Autodesk Inventor part; units mm, degrees
(part 2 of 15)
  arc A531 (-9.765, -99.9538) -> (-9.765, -99.8522) centre (-9.765, -99.903) ccw
  arc A532 (-11.035, -99.8522) -> (-11.035, -99.9538) centre (-11.035, -99.903) ccw
  arc A533 (-23.984, 46.0572) -> (-23.984, 46.1588) centre (-23.984, 46.108) ccw
  line L129 (-17.235, -109.297) -> (-17.235, -106.503)
  arc A534 (-17.1842, -106.503) -> (-17.2858, -106.503) centre (-17.235, -106.503) ccw
  arc A535 (-17.2858, -109.297) -> (-17.1842, -109.297) centre (-17.235, -109.297) ccw
  line L130 (-17.235, -106.503) -> (-15.965, -106.503)
  arc A536 (-15.965, -106.5538) -> (-15.965, -106.4522) centre (-15.965, -106.503) ccw
  arc A537 (-17.235, -106.4522) -> (-17.235, -106.5538) centre (-17.235, -106.503) ccw
  line L131 (-15.965, -106.503) -> (-15.965, -109.297)
  arc A538 (-16.0158, -109.297) -> (-15.9142, -109.297) centre (-15.965, -109.297) ccw
  arc A539 (-15.9142, -106.503) -> (-16.0158, -106.503) centre (-15.965, -106.503) ccw
  line L132 (-15.965, -109.297) -> (-17.235, -109.297)
  arc A540 (-17.235, -109.2462) -> (-17.235, -109.3478) centre (-17.235, -109.297) ccw
  arc A541 (-15.965, -109.3478) -> (-15.965, -109.2462) centre (-15.965, -109.297) ccw
  arc A542 (-26.016, 46.1588) -> (-26.016, 46.0572) centre (-26.016, 46.108) ccw
  line L133 (-15.808, -109.416) -> (-15.808, -107.384)
  arc A543 (-15.7572, -107.384) -> (-15.8588, -107.384) centre (-15.808, -107.384) ccw
  arc A544 (-15.8588, -109.416) -> (-15.7572, -109.416) centre (-15.808, -109.416) ccw
  line L134 (-15.808, -107.384) -> (-14.792, -107.384)
  arc A545 (-14.792, -107.4348) -> (-14.792, -107.3332) centre (-14.792, -107.384) ccw
  arc A546 (-15.808, -107.3332) -> (-15.808, -107.4348) centre (-15.808, -107.384) ccw
  line L135 (-14.792, -107.384) -> (-14.792, -109.416)
  arc A547 (-14.8428, -109.416) -> (-14.7412, -109.416) centre (-14.792, -109.416) ccw
  arc A548 (-14.7412, -107.384) -> (-14.8428, -107.384) centre (-14.792, -107.384) ccw
  line L136 (-14.792, -109.416) -> (-15.808, -109.416)
  arc A549 (-15.808, -109.3652) -> (-15.808, -109.4668) centre (-15.808, -109.416) ccw
  arc A550 (-14.792, -109.4668) -> (-14.792, -109.3652) centre (-14.792, -109.416) ccw
  line L137 (-23.984, 46.108) -> (-23.984, 45.092)
  line L138 (9.757, -79.0892) -> (9.757, -74.1108)
  arc A551 (9.8078, -74.1108) -> (9.7062, -74.1108) centre (9.757, -74.1108) ccw
  arc A552 (9.7062, -79.0892) -> (9.8078, -79.0892) centre (9.757, -79.0892) ccw
  line L139 (9.757, -74.1108) -> (12.043, -74.1108)
  arc A553 (12.043, -74.1616) -> (12.043, -74.06) centre (12.043, -74.1108) ccw
  arc A554 (9.757, -74.06) -> (9.757, -74.1616) centre (9.757, -74.1108) ccw
  line L140 (12.043, -74.1108) -> (12.043, -79.0892)
  arc A555 (11.9922, -79.0892) -> (12.0938, -79.0892) centre (12.043, -79.0892) ccw
  arc A556 (12.0938, -74.1108) -> (11.9922, -74.1108) centre (12.043, -74.1108) ccw
  line L141 (12.043, -79.0892) -> (9.757, -79.0892)
  arc A557 (9.757, -79.0384) -> (9.757, -79.14) centre (9.757, -79.0892) ccw
  arc A558 (12.043, -79.14) -> (12.043, -79.0384) centre (12.043, -79.0892) ccw
  arc A559 (-24.0348, 45.092) -> (-23.9332, 45.092) centre (-23.984, 45.092) ccw
  line L142 (9.203, -79.065) -> (11.997, -79.065)
  arc A560 (11.997, -79.1158) -> (11.997, -79.0142) centre (11.997, -79.065) ccw
  arc A561 (9.203, -79.0142) -> (9.203, -79.1158) centre (9.203, -79.065) ccw
  line L143 (11.997, -79.065) -> (11.997, -80.335)
  arc A562 (11.9462, -80.335) -> (12.0478, -80.335) centre (11.997, -80.335) ccw
  arc A563 (12.0478, -79.065) -> (11.9462, -79.065) centre (11.997, -79.065) ccw
  line L144 (11.997, -80.335) -> (9.203, -80.335)
  arc A564 (9.203, -80.2842) -> (9.203, -80.3858) centre (9.203, -80.335) ccw
  arc A565 (11.997, -80.3858) -> (11.997, -80.2842) centre (11.997, -80.335) ccw
  line L145 (9.203, -80.335) -> (9.203, -79.065)
  arc A566 (9.2538, -79.065) -> (9.1522, -79.065) centre (9.203, -79.065) ccw
  arc A567 (9.1522, -80.335) -> (9.2538, -80.335) centre (9.203, -80.335) ccw
  arc A568 (-23.9332, 46.108) -> (-24.0348, 46.108) centre (-23.984, 46.108) ccw
  line L146 (8.165, -77.997) -> (8.165, -75.203)
  arc A569 (8.2158, -75.203) -> (8.1142, -75.203) centre (8.165, -75.203) ccw
  arc A570 (8.1142, -77.997) -> (8.2158, -77.997) centre (8.165, -77.997) ccw
  line L147 (8.165, -75.203) -> (9.435, -75.203)
  arc A571 (9.435, -75.2538) -> (9.435, -75.1522) centre (9.435, -75.203) ccw
  arc A572 (8.165, -75.1522) -> (8.165, -75.2538) centre (8.165, -75.203) ccw
  line L148 (9.435, -75.203) -> (9.435, -77.997)
  arc A573 (9.3842, -77.997) -> (9.4858, -77.997) centre (9.435, -77.997) ccw
  arc A574 (9.4858, -75.203) -> (9.3842, -75.203) centre (9.435, -75.203) ccw
  line L149 (9.435, -77.997) -> (8.165, -77.997)
  arc A575 (8.165, -77.9462) -> (8.165, -78.0478) centre (8.165, -77.997) ccw
  arc A576 (9.435, -78.0478) -> (9.435, -77.9462) centre (9.435, -77.997) ccw
  line L150 (-23.984, 45.092) -> (-26.016, 45.092)
  line L151 (9.584, -83.992) -> (11.616, -83.992)
  arc A577 (11.616, -84.0428) -> (11.616, -83.9412) centre (11.616, -83.992) ccw
  arc A578 (9.584, -83.9412) -> (9.584, -84.0428) centre (9.584, -83.992) ccw
  line L152 (11.616, -83.992) -> (11.616, -85.008)
  arc A579 (11.5652, -85.008) -> (11.6668, -85.008) centre (11.616, -85.008) ccw
  arc A580 (11.6668, -83.992) -> (11.5652, -83.992) centre (11.616, -83.992) ccw
  line L153 (11.616, -85.008) -> (9.584, -85.008)
  arc A581 (9.584, -84.9572) -> (9.584, -85.0588) centre (9.584, -85.008) ccw
  arc A582 (11.616, -85.0588) -> (11.616, -84.9572) centre (11.616, -85.008) ccw
  line L154 (9.584, -85.008) -> (9.584, -83.992)
  arc A583 (9.6348, -83.992) -> (9.5332, -83.992) centre (9.584, -83.992) ccw
  arc A584 (9.5332, -85.008) -> (9.6348, -85.008) centre (9.584, -85.008) ccw
  arc A585 (-26.016, 45.1428) -> (-26.016, 45.0412) centre (-26.016, 45.092) ccw
  line L155 (12.365, -77.997) -> (12.365, -75.203)
  arc A586 (12.4158, -75.203) -> (12.3142, -75.203) centre (12.365, -75.203) ccw
  arc A587 (12.3142, -77.997) -> (12.4158, -77.997) centre (12.365, -77.997) ccw
  line L156 (12.365, -75.203) -> (13.635, -75.203)
  arc A588 (13.635, -75.2538) -> (13.635, -75.1522) centre (13.635, -75.203) ccw
  arc A589 (12.365, -75.1522) -> (12.365, -75.2538) centre (12.365, -75.203) ccw
  line L157 (13.635, -75.203) -> (13.635, -77.997)
  arc A590 (13.5842, -77.997) -> (13.6858, -77.997) centre (13.635, -77.997) ccw
  arc A591 (13.6858, -75.203) -> (13.5842, -75.203) centre (13.635, -75.203) ccw
  line L158 (13.635, -77.997) -> (12.365, -77.997)
  arc A592 (12.365, -77.9462) -> (12.365, -78.0478) centre (12.365, -77.997) ccw
  arc A593 (13.635, -78.0478) -> (13.635, -77.9462) centre (13.635, -77.997) ccw
  arc A594 (-23.984, 45.0412) -> (-23.984, 45.1428) centre (-23.984, 45.092) ccw
  line L159 (13.765, -77.997) -> (13.765, -75.203)
  arc A595 (13.8158, -75.203) -> (13.7142, -75.203) centre (13.765, -75.203) ccw
  arc A596 (13.7142, -77.997) -> (13.8158, -77.997) centre (13.765, -77.997) ccw
  line L160 (13.765, -75.203) -> (15.035, -75.203)
  arc A597 (15.035, -75.2538) -> (15.035, -75.1522) centre (15.035, -75.203) ccw
  arc A598 (13.765, -75.1522) -> (13.765, -75.2538) centre (13.765, -75.203) ccw
  line L161 (15.035, -75.203) -> (15.035, -77.997)
  arc A599 (14.9842, -77.997) -> (15.0858, -77.997) centre (15.035, -77.997) ccw
  arc A600 (15.0858, -75.203) -> (14.9842, -75.203) centre (15.035, -75.203) ccw
  line L162 (15.035, -77.997) -> (13.765, -77.997)
  arc A601 (13.765, -77.9462) -> (13.765, -78.0478) centre (13.765, -77.997) ccw
  arc A602 (15.035, -78.0478) -> (15.035, -77.9462) centre (15.035, -77.997) ccw
  line L163 (-26.016, 45.092) -> (-26.016, 46.108)
  line L164 (15.165, -77.997) -> (15.165, -75.203)
  arc A603 (15.2158, -75.203) -> (15.1142, -75.203) centre (15.165, -75.203) ccw
  arc A604 (15.1142, -77.997) -> (15.2158, -77.997) centre (15.165, -77.997) ccw
  line L165 (15.165, -75.203) -> (16.435, -75.203)
  arc A605 (16.435, -75.2538) -> (16.435, -75.1522) centre (16.435, -75.203) ccw
  arc A606 (15.165, -75.1522) -> (15.165, -75.2538) centre (15.165, -75.203) ccw
  line L166 (16.435, -75.203) -> (16.435, -77.997)
  arc A607 (16.3842, -77.997) -> (16.4858, -77.997) centre (16.435, -77.997) ccw
  arc A608 (16.4858, -75.203) -> (16.3842, -75.203) centre (16.435, -75.203) ccw
  line L167 (16.435, -77.997) -> (15.165, -77.997)
  arc A609 (15.165, -77.9462) -> (15.165, -78.0478) centre (15.165, -77.997) ccw
  arc A610 (16.435, -78.0478) -> (16.435, -77.9462) centre (16.435, -77.997) ccw
  arc A611 (-25.9652, 46.108) -> (-26.0668, 46.108) centre (-26.016, 46.108) ccw
  line L168 (-17, 38.5) -> (-17, 36.9)
  arc A612 (-17.0318, 36.9) -> (-16.9683, 36.9) centre (-17.0001, 36.9) ccw
  arc A613 (-16.9683, 38.5) -> (-17.0318, 38.5) centre (-17.0001, 38.5) ccw
  line L169 (-17, 36.9) -> (-17.8, 36.9)
  arc A614 (-17.8, 36.9317) -> (-17.8, 36.8683) centre (-17.8, 36.9) ccw
  arc A615 (-17, 36.8683) -> (-17, 36.9317) centre (-17, 36.9) ccw
  line L170 (-17.8, 38.5) -> (-17, 38.5)
  arc A616 (-17, 38.4683) -> (-17, 38.5317) centre (-17, 38.5) ccw
  arc A617 (-17.8, 38.5317) -> (-17.8, 38.4683) centre (-17.8, 38.5) ccw
  line L171 (-17.8, 36.9) -> (-17.8, 38.5)
  arc A618 (-17.7682, 38.5) -> (-17.8318, 38.5) centre (-17.8, 38.5) ccw
  arc A619 (-17.8318, 36.9) -> (-17.7682, 36.9) centre (-17.8, 36.9) ccw
  arc A620 (-26.0668, 45.092) -> (-25.9652, 45.092) centre (-26.016, 45.092) ccw
  line L172 (-22.8, -4.4) -> (-21.2, -4.4)
  arc A621 (-21.2, -4.4317) -> (-21.2, -4.3682) centre (-21.2, -4.4) ccw
  arc A622 (-22.8, -4.3682) -> (-22.8, -4.4317) centre (-22.8, -4.4) ccw
  line L173 (-21.2, -4.4) -> (-21.2, -5.2)
  arc A623 (-21.2317, -5.2) -> (-21.1682, -5.2) centre (-21.2, -5.2) ccw
  arc A624 (-21.1682, -4.4) -> (-21.2317, -4.4) centre (-21.2, -4.4) ccw
  line L174 (-22.8, -5.2) -> (-22.8, -4.4)
  arc A625 (-22.7682, -4.4) -> (-22.8318, -4.4) centre (-22.8, -4.4) ccw
  arc A626 (-22.8318, -5.2) -> (-22.7682, -5.2) centre (-22.8, -5.2) ccw
  line L175 (-21.2, -5.2) -> (-22.8, -5.2)
  arc A627 (-22.8, -5.1682) -> (-22.8, -5.2317) centre (-22.8, -5.2) ccw
  arc A628 (-21.2, -5.2317) -> (-21.2, -5.1682) centre (-21.2, -5.2) ccw
  line L176 (-26.016, 48.108) -> (-23.984, 48.108)
  line L177 (17.7, -53) -> (17.7, -51.4)
  arc A629 (17.7318, -51.4) -> (17.6682, -51.4) centre (17.7, -51.4) ccw
  arc A630 (17.6682, -53) -> (17.7318, -53) centre (17.7, -53) ccw
  line L178 (17.7, -51.4) -> (18.5, -51.4)
  arc A631 (18.5, -51.4317) -> (18.5, -51.3682) centre (18.5, -51.4) ccw
  arc A632 (17.7, -51.3682) -> (17.7, -51.4317) centre (17.7, -51.4) ccw
  line L179 (18.5, -53) -> (17.7, -53)
  arc A633 (17.7, -52.9682) -> (17.7, -53.0317) centre (17.7, -53) ccw
  arc A634 (18.5, -53.0317) -> (18.5, -52.9682) centre (18.5, -53) ccw
  line L180 (18.5, -51.4) -> (18.5, -53)
  arc A635 (18.4683, -53) -> (18.5318, -53) centre (18.5, -53) ccw
  arc A636 (18.5318, -51.4) -> (18.4683, -51.4) centre (18.5, -51.4) ccw
  arc A637 (-23.984, 48.0572) -> (-23.984, 48.1588) centre (-23.984, 48.108) ccw
  line L181 (-19.9, 38.5) -> (-19.9, 40.1)
  arc A638 (-19.8682, 40.1) -> (-19.9317, 40.1) centre (-19.9, 40.1) ccw
  arc A639 (-19.9317, 38.5) -> (-19.8682, 38.5) centre (-19.9, 38.5) ccw
  line L182 (-19.9, 40.1) -> (-19.1, 40.1)
  arc A640 (-19.1, 40.0683) -> (-19.1, 40.1318) centre (-19.1, 40.1) ccw
  arc A641 (-19.9, 40.1318) -> (-19.9, 40.0683) centre (-19.9, 40.1) ccw
  line L183 (-19.1, 38.5) -> (-19.9, 38.5)
  arc A642 (-19.9, 38.5317) -> (-19.9, 38.4683) centre (-19.9, 38.5) ccw
  arc A643 (-19.1, 38.4683) -> (-19.1, 38.5317) centre (-19.1, 38.5) ccw
  line L184 (-19.1, 40.1) -> (-19.1, 38.5)
  arc A644 (-19.1317, 38.5) -> (-19.0682, 38.5) centre (-19.1, 38.5) ccw
  arc A645 (-19.0682, 40.1) -> (-19.1317, 40.1) centre (-19.1, 40.1) ccw
  arc A646 (-26.016, 48.1588) -> (-26.016, 48.0572) centre (-26.016, 48.108) ccw
  line L185 (-19.6, 7) -> (-19.6, 5.4)
  arc A647 (-19.6317, 5.4) -> (-19.5682, 5.4) centre (-19.6, 5.4) ccw
  arc A648 (-19.5682, 7) -> (-19.6317, 7) centre (-19.6, 7) ccw
  line L186 (-19.6, 5.4) -> (-20.4, 5.4)
  arc A649 (-20.4, 5.4317) -> (-20.4, 5.3683) centre (-20.4, 5.4) ccw
  arc A650 (-19.6, 5.3683) -> (-19.6, 5.4317) centre (-19.6, 5.4) ccw
  line L187 (-20.4, 7) -> (-19.6, 7)
  arc A651 (-19.6, 6.9683) -> (-19.6, 7.0317) centre (-19.6, 7) ccw
  arc A652 (-20.4, 7.0317) -> (-20.4, 6.9683) centre (-20.4, 7) ccw
  line L188 (-20.4, 5.4) -> (-20.4, 7)
  arc A653 (-20.3682, 7) -> (-20.4317, 7) centre (-20.4, 7) ccw
  arc A654 (-20.4317, 5.4) -> (-20.3682, 5.4) centre (-20.4, 5.4) ccw
  line L189 (-23.984, 48.108) -> (-23.984, 47.092)
  line L190 (-5.6, 8) -> (-5.6, 6.4)
  arc A655 (-5.6317, 6.4) -> (-5.5682, 6.4) centre (-5.6, 6.4) ccw
  arc A656 (-5.5682, 8) -> (-5.6317, 8) centre (-5.6, 8) ccw
  line L191 (-5.6, 6.4) -> (-6.4, 6.4)
  arc A657 (-6.4, 6.4317) -> (-6.4, 6.3683) centre (-6.4, 6.4) ccw
  arc A658 (-5.6, 6.3683) -> (-5.6, 6.4317) centre (-5.6, 6.4) ccw
  line L192 (-6.4, 8) -> (-5.6, 8)
  arc A659 (-5.6, 7.9683) -> (-5.6, 8.0317) centre (-5.6, 8) ccw
  arc A660 (-6.4, 8.0317) -> (-6.4, 7.9683) centre (-6.4, 8) ccw
  line L193 (-6.4, 6.4) -> (-6.4, 8)
  arc A661 (-6.3682, 8) -> (-6.4317, 8) centre (-6.4, 8) ccw
  arc A662 (-6.4317, 6.4) -> (-6.3682, 6.4) centre (-6.4, 6.4) ccw
  arc A663 (-24.0348, 47.092) -> (-23.9332, 47.092) centre (-23.984, 47.092) ccw
  line L194 (20.908, -110.784) -> (20.908, -112.816)
  arc A664 (20.8572, -112.816) -> (20.9588, -112.816) centre (20.908, -112.816) ccw
  arc A665 (20.9588, -110.784) -> (20.8572, -110.784) centre (20.908, -110.784) ccw
  line L195 (20.908, -112.816) -> (19.892, -112.816)
  arc A666 (19.892, -112.7652) -> (19.892, -112.8668) centre (19.892, -112.816) ccw
  arc A667 (20.908, -112.8668) -> (20.908, -112.7652) centre (20.908, -112.816) ccw
  line L196 (19.892, -112.816) -> (19.892, -110.784)
  arc A668 (19.9428, -110.784) -> (19.8412, -110.784) centre (19.892, -110.784) ccw
  arc A669 (19.8412, -112.816) -> (19.9428, -112.816) centre (19.892, -112.816) ccw
  line L197 (19.892, -110.784) -> (20.908, -110.784)
  arc A670 (20.908, -110.8348) -> (20.908, -110.7332) centre (20.908, -110.784) ccw
  arc A671 (19.892, -110.7332) -> (19.892, -110.8348) centre (19.892, -110.784) ccw
  arc A672 (-23.9332, 48.108) -> (-24.0348, 48.108) centre (-23.984, 48.108) ccw
  line L198 (19.892, -116.216) -> (19.892, -114.184)
  arc A673 (19.9428, -114.184) -> (19.8412, -114.184) centre (19.892, -114.184) ccw
  arc A674 (19.8412, -116.216) -> (19.9428, -116.216) centre (19.892, -116.216) ccw
  line L199 (19.892, -114.184) -> (20.908, -114.184)
  arc A675 (20.908, -114.2348) -> (20.908, -114.1332) centre (20.908, -114.184) ccw
  arc A676 (19.892, -114.1332) -> (19.892, -114.2348) centre (19.892, -114.184) ccw
  line L200 (20.908, -114.184) -> (20.908, -116.216)
  arc A677 (20.8572, -116.216) -> (20.9588, -116.216) centre (20.908, -116.216) ccw
  arc A678 (20.9588, -114.184) -> (20.8572, -114.184) centre (20.908, -114.184) ccw
  line L201 (20.908, -116.216) -> (19.892, -116.216)
  arc A679 (19.892, -116.1652) -> (19.892, -116.2668) centre (19.892, -116.216) ccw
  arc A680 (20.908, -116.2668) -> (20.908, -116.1652) centre (20.908, -116.216) ccw
  line L202 (-23.984, 47.092) -> (-26.016, 47.092)
  line L203 (13.184, -105.892) -> (15.216, -105.892)
  arc A681 (15.216, -105.9428) -> (15.216, -105.8412) centre (15.216, -105.892) ccw
  arc A682 (13.184, -105.8412) -> (13.184, -105.9428) centre (13.184, -105.892) ccw
  line L204 (15.216, -105.892) -> (15.216, -106.908)
  arc A683 (15.1652, -106.908) -> (15.2668, -106.908) centre (15.216, -106.908) ccw
  arc A684 (15.2668, -105.892) -> (15.1652, -105.892) centre (15.216, -105.892) ccw
  line L205 (15.216, -106.908) -> (13.184, -106.908)
  arc A685 (13.184, -106.8572) -> (13.184, -106.9588) centre (13.184, -106.908) ccw
  arc A686 (15.216, -106.9588) -> (15.216, -106.8572) centre (15.216, -106.908) ccw
  line L206 (13.184, -106.908) -> (13.184, -105.892)
  arc A687 (13.2348, -105.892) -> (13.1332, -105.892) centre (13.184, -105.892) ccw
  arc A688 (13.1332, -106.908) -> (13.2348, -106.908) centre (13.184, -106.908) ccw
  arc A689 (-26.016, 47.1428) -> (-26.016, 47.0412) centre (-26.016, 47.092) ccw
  line L207 (7.384, -108.092) -> (9.416, -108.092)
  arc A690 (9.416, -108.1428) -> (9.416, -108.0412) centre (9.416, -108.092) ccw
  arc A691 (7.384, -108.0412) -> (7.384, -108.1428) centre (7.384, -108.092) ccw
  line L208 (9.416, -108.092) -> (9.416, -109.108)
  arc A692 (9.3652, -109.108) -> (9.4668, -109.108) centre (9.416, -109.108) ccw
  arc A693 (9.4668, -108.092) -> (9.3652, -108.092) centre (9.416, -108.092) ccw
  line L209 (9.416, -109.108) -> (7.384, -109.108)
  arc A694 (7.384, -109.0572) -> (7.384, -109.1588) centre (7.384, -109.108) ccw
  arc A695 (9.416, -109.1588) -> (9.416, -109.0572) centre (9.416, -109.108) ccw
  line L210 (7.384, -109.108) -> (7.384, -108.092)
  arc A696 (7.4348, -108.092) -> (7.3332, -108.092) centre (7.384, -108.092) ccw
  arc A697 (7.3332, -109.108) -> (7.4348, -109.108) centre (7.384, -109.108) ccw
  arc A698 (-23.984, 47.0412) -> (-23.984, 47.1428) centre (-23.984, 47.092) ccw
  line L211 (9.408, -106.084) -> (9.408, -108.116)
  arc A699 (9.3572, -108.116) -> (9.4588, -108.116) centre (9.408, -108.116) ccw
  arc A700 (9.4588, -106.084) -> (9.3572, -106.084) centre (9.408, -106.084) ccw
  line L212 (9.408, -108.116) -> (8.392, -108.116)
  arc A701 (8.392, -108.0652) -> (8.392, -108.1668) centre (8.392, -108.116) ccw
  arc A702 (9.408, -108.1668) -> (9.408, -108.0652) centre (9.408, -108.116) ccw
  line L213 (8.392, -108.116) -> (8.392, -106.084)
  arc A703 (8.4428, -106.084) -> (8.3412, -106.084) centre (8.392, -106.084) ccw
  arc A704 (8.3412, -108.116) -> (8.4428, -108.116) centre (8.392, -108.116) ccw
  line L214 (8.392, -106.084) -> (9.408, -106.084)
  arc A705 (9.408, -106.1348) -> (9.408, -106.0332) centre (9.408, -106.084) ccw
  arc A706 (8.392, -106.0332) -> (8.392, -106.1348) centre (8.392, -106.084) ccw
  line L215 (-26.016, 47.092) -> (-26.016, 48.108)
  line L216 (-8.416, -106.092) -> (-6.384, -106.092)
  arc A707 (-6.384, -106.1428) -> (-6.384, -106.0412) centre (-6.384, -106.092) ccw
  arc A708 (-8.416, -106.0412) -> (-8.416, -106.1428) centre (-8.416, -106.092) ccw
  line L217 (-6.384, -106.092) -> (-6.384, -107.108)
  arc A709 (-6.4348, -107.108) -> (-6.3332, -107.108) centre (-6.384, -107.108) ccw
  arc A710 (-6.3332, -106.092) -> (-6.4348, -106.092) centre (-6.384, -106.092) ccw
  line L218 (-6.384, -107.108) -> (-8.416, -107.108)
  arc A711 (-8.416, -107.0572) -> (-8.416, -107.1588) centre (-8.416, -107.108) ccw
  arc A712 (-6.384, -107.1588) -> (-6.384, -107.0572) centre (-6.384, -107.108) ccw
  line L219 (-8.416, -107.108) -> (-8.416, -106.092)
  arc A713 (-8.3652, -106.092) -> (-8.4668, -106.092) centre (-8.416, -106.092) ccw
  arc A714 (-8.4668, -107.108) -> (-8.3652, -107.108) centre (-8.416, -107.108) ccw
  arc A715 (-25.9652, 48.108) -> (-26.0668, 48.108) centre (-26.016, 48.108) ccw
  line L220 (13.335, -97.103) -> (13.335, -99.897)
  arc A716 (13.2842, -99.897) -> (13.3858, -99.897) centre (13.335, -99.897) ccw
  arc A717 (13.3858, -97.103) -> (13.2842, -97.103) centre (13.335, -97.103) ccw
  line L221 (13.335, -99.897) -> (12.065, -99.897)
  arc A718 (12.065, -99.8462) -> (12.065, -99.9478) centre (12.065, -99.897) ccw
  arc A719 (13.335, -99.9478) -> (13.335, -99.8462) centre (13.335, -99.897) ccw
  line L222 (12.065, -99.897) -> (12.065, -97.103)
  arc A720 (12.1158, -97.103) -> (12.0142, -97.103) centre (12.065, -97.103) ccw
  arc A721 (12.0142, -99.897) -> (12.1158, -99.897) centre (12.065, -99.897) ccw
  line L223 (12.065, -97.103) -> (13.335, -97.103)
  arc A722 (13.335, -97.1538) -> (13.335, -97.0522) centre (13.335, -97.103) ccw
  arc A723 (12.065, -97.0522) -> (12.065, -97.1538) centre (12.065, -97.103) ccw
  arc A724 (-26.0668, 47.092) -> (-25.9652, 47.092) centre (-26.016, 47.092) ccw
  line L224 (12.192, -103.816) -> (12.192, -101.784)
  arc A725 (12.2428, -101.784) -> (12.1412, -101.784) centre (12.192, -101.784) ccw
  arc A726 (12.1412, -103.816) -> (12.2428, -103.816) centre (12.192, -103.816) ccw
  line L225 (12.192, -101.784) -> (13.208, -101.784)
  arc A727 (13.208, -101.8348) -> (13.208, -101.7332) centre (13.208, -101.784) ccw
  arc A728 (12.192, -101.7332) -> (12.192, -101.8348) centre (12.192, -101.784) ccw
  line L226 (13.208, -101.784) -> (13.208, -103.816)
  arc A729 (13.1572, -103.816) -> (13.2588, -103.816) centre (13.208, -103.816) ccw
  arc A730 (13.2588, -101.784) -> (13.1572, -101.784) centre (13.208, -101.784) ccw
  line L227 (13.208, -103.816) -> (12.192, -103.816)
  arc A731 (12.192, -103.7652) -> (12.192, -103.8668) centre (12.192, -103.816) ccw
  arc A732 (13.208, -103.8668) -> (13.208, -103.7652) centre (13.208, -103.816) ccw
  line L228 (-26.016, 44.108) -> (-23.984, 44.108)
  line L229 (12.135, -104.003) -> (12.135, -106.797)
  arc A733 (12.0842, -106.797) -> (12.1858, -106.797) centre (12.135, -106.797) ccw
  arc A734 (12.1858, -104.003) -> (12.0842, -104.003) centre (12.135, -104.003) ccw
  line L230 (12.135, -106.797) -> (10.865, -106.797)
  arc A735 (10.865, -106.7462) -> (10.865, -106.8478) centre (10.865, -106.797) ccw
  arc A736 (12.135, -106.8478) -> (12.135, -106.7462) centre (12.135, -106.797) ccw
  line L231 (10.865, -106.797) -> (10.865, -104.003)
  arc A737 (10.9158, -104.003) -> (10.8142, -104.003) centre (10.865, -104.003) ccw
  arc A738 (10.8142, -106.797) -> (10.9158, -106.797) centre (10.865, -106.797) ccw
  line L232 (10.865, -104.003) -> (12.135, -104.003)
  arc A739 (12.135, -104.0538) -> (12.135, -103.9522) centre (12.135, -104.003) ccw
  arc A740 (10.865, -103.9522) -> (10.865, -104.0538) centre (10.865, -104.003) ccw
  arc A741 (-23.984, 44.0572) -> (-23.984, 44.1588) centre (-23.984, 44.108) ccw
  line L233 (14.216, -105.808) -> (12.184, -105.808)
  arc A742 (12.184, -105.7572) -> (12.184, -105.8588) centre (12.184, -105.808) ccw
  arc A743 (14.216, -105.8588) -> (14.216, -105.7572) centre (14.216, -105.808) ccw
  line L234 (12.184, -105.808) -> (12.184, -104.792)
  arc A744 (12.2348, -104.792) -> (12.1332, -104.792) centre (12.184, -104.792) ccw
  arc A745 (12.1332, -105.808) -> (12.2348, -105.808) centre (12.184, -105.808) ccw
  line L235 (12.184, -104.792) -> (14.216, -104.792)
  arc A746 (14.216, -104.8428) -> (14.216, -104.7412) centre (14.216, -104.792) ccw
  arc A747 (12.184, -104.7412) -> (12.184, -104.8428) centre (12.184, -104.792) ccw
  line L236 (14.216, -104.792) -> (14.216, -105.808)
  arc A748 (14.1652, -105.808) -> (14.2668, -105.808) centre (14.216, -105.808) ccw
  arc A749 (14.2668, -104.792) -> (14.1652, -104.792) centre (14.216, -104.792) ccw
  arc A750 (-26.016, 44.1588) -> (-26.016, 44.0572) centre (-26.016, 44.108) ccw
  line L237 (-5.392, -107.084) -> (-5.392, -109.116)
  arc A751 (-5.4428, -109.116) -> (-5.3412, -109.116) centre (-5.392, -109.116) ccw
  arc A752 (-5.3412, -107.084) -> (-5.4428, -107.084) centre (-5.392, -107.084) ccw
  line L238 (-5.392, -109.116) -> (-6.408, -109.116)
  arc A753 (-6.408, -109.0652) -> (-6.408, -109.1668) centre (-6.408, -109.116) ccw
  arc A754 (-5.392, -109.1668) -> (-5.392, -109.0652) centre (-5.392, -109.116) ccw
  line L239 (-6.408, -109.116) -> (-6.408, -107.084)
  arc A755 (-6.3572, -107.084) -> (-6.4588, -107.084) centre (-6.408, -107.084) ccw
  arc A756 (-6.4588, -109.116) -> (-6.3572, -109.116) centre (-6.408, -109.116) ccw
  line L240 (-6.408, -107.084) -> (-5.392, -107.084)
  arc A757 (-5.392, -107.1348) -> (-5.392, -107.0332) centre (-5.392, -107.084) ccw
  arc A758 (-6.408, -107.0332) -> (-6.408, -107.1348) centre (-6.408, -107.084) ccw
  line L241 (-23.984, 44.108) -> (-23.984, 43.092)
  line L242 (-3.384, -109.108) -> (-5.416, -109.108)
  arc A759 (-5.416, -109.0572) -> (-5.416, -109.1588) centre (-5.416, -109.108) ccw
  arc A760 (-3.384, -109.1588) -> (-3.384, -109.0572) centre (-3.384, -109.108) ccw
  line L243 (-5.416, -109.108) -> (-5.416, -108.092)
  arc A761 (-5.3652, -108.092) -> (-5.4668, -108.092) centre (-5.416, -108.092) ccw
  arc A762 (-5.4668, -109.108) -> (-5.3652, -109.108) centre (-5.416, -109.108) ccw
  line L244 (-5.416, -108.092) -> (-3.384, -108.092)
  arc A763 (-3.384, -108.1428) -> (-3.384, -108.0412) centre (-3.384, -108.092) ccw
  arc A764 (-5.416, -108.0412) -> (-5.416, -108.1428) centre (-5.416, -108.092) ccw
  line L245 (-3.384, -108.092) -> (-3.384, -109.108)
  arc A765 (-3.4348, -109.108) -> (-3.3332, -109.108) centre (-3.384, -109.108) ccw
  arc A766 (-3.3332, -108.092) -> (-3.4348, -108.092) centre (-3.384, -108.092) ccw
  arc A767 (-24.0348, 43.092) -> (-23.9332, 43.092) centre (-23.984, 43.092) ccw
  line L246 (16.216, -101.808) -> (14.184, -101.808)
  arc A768 (14.184, -101.7572) -> (14.184, -101.8588) centre (14.184, -101.808) ccw
  arc A769 (16.216, -101.8588) -> (16.216, -101.7572) centre (16.216, -101.808) ccw
  line L247 (14.184, -101.808) -> (14.184, -100.792)
  arc A770 (14.2348, -100.792) -> (14.1332, -100.792) centre (14.184, -100.792) ccw
  arc A771 (14.1332, -101.808) -> (14.2348, -101.808) centre (14.184, -101.808) ccw
  line L248 (14.184, -100.792) -> (16.216, -100.792)
  arc A772 (16.216, -100.8428) -> (16.216, -100.7412) centre (16.216, -100.792) ccw
  arc A773 (14.184, -100.7412) -> (14.184, -100.8428) centre (14.184, -100.792) ccw
  line L249 (16.216, -100.792) -> (16.216, -101.808)
  arc A774 (16.1652, -101.808) -> (16.2668, -101.808) centre (16.216, -101.808) ccw
  arc A775 (16.2668, -100.792) -> (16.1652, -100.792) centre (16.216, -100.792) ccw
  arc A776 (-23.9332, 44.108) -> (-24.0348, 44.108) centre (-23.984, 44.108) ccw
  line L250 (16.216, -103.808) -> (14.184, -103.808)
  arc A777 (14.184, -103.7572) -> (14.184, -103.8588) centre (14.184, -103.808) ccw
  arc A778 (16.216, -103.8588) -> (16.216, -103.7572) centre (16.216, -103.808) ccw
  line L251 (14.184, -103.808) -> (14.184, -102.792)
  arc A779 (14.2348, -102.792) -> (14.1332, -102.792) centre (14.184, -102.792) ccw
  arc A780 (14.1332, -103.808) -> (14.2348, -103.808) centre (14.184, -103.808) ccw
  line L252 (14.184, -102.792) -> (16.216, -102.792)
  arc A781 (16.216, -102.8428) -> (16.216, -102.7412) centre (16.216, -102.792) ccw
  arc A782 (14.184, -102.7412) -> (14.184, -102.8428) centre (14.184, -102.792) ccw
  line L253 (16.216, -102.792) -> (16.216, -103.808)
  arc A783 (16.1652, -103.808) -> (16.2668, -103.808) centre (16.216, -103.808) ccw
  arc A784 (16.2668, -102.792) -> (16.1652, -102.792) centre (16.216, -102.792) ccw
  line L254 (-23.984, 43.092) -> (-26.016, 43.092)
  line L255 (-6.911, 46.3542) -> (-6.911, 42.6458)
  arc A785 (-6.9618, 42.6458) -> (-6.8602, 42.6458) centre (-6.911, 42.6458) ccw
  arc A786 (-6.8602, 46.3542) -> (-6.9618, 46.3542) centre (-6.911, 46.3542) ccw
  line L256 (-6.911, 42.6458) -> (-8.689, 42.6458)
  arc A787 (-8.689, 42.6966) -> (-8.689, 42.595) centre (-8.689, 42.6458) ccw
  arc A788 (-6.911, 42.595) -> (-6.911, 42.6966) centre (-6.911, 42.6458) ccw
  line L257 (-8.689, 42.6458) -> (-8.689, 46.3542)
  arc A789 (-8.6382, 46.3542) -> (-8.7398, 46.3542) centre (-8.689, 46.3542) ccw
  arc A790 (-8.7398, 42.6458) -> (-8.6382, 42.6458) centre (-8.689, 42.6458) ccw
  line L258 (-8.689, 46.3542) -> (-6.911, 46.3542)
  arc A791 (-6.911, 46.3034) -> (-6.911, 46.405) centre (-6.911, 46.3542) ccw
  arc A792 (-8.689, 46.405) -> (-8.689, 46.3034) centre (-8.689, 46.3542) ccw
  arc A793 (-26.016, 43.1428) -> (-26.016, 43.0412) centre (-26.016, 43.092) ccw
  line L259 (-11.489, 41.9458) -> (-11.489, 45.6542)
  arc A794 (-11.4382, 45.6542) -> (-11.5398, 45.6542) centre (-11.489, 45.6542) ccw
  arc A795 (-11.5398, 41.9458) -> (-11.4382, 41.9458) centre (-11.489, 41.9458) ccw
  line L260 (-11.489, 45.6542) -> (-9.711, 45.6542)
  arc A796 (-9.711, 45.6034) -> (-9.711, 45.705) centre (-9.711, 45.6542) ccw
  arc A797 (-11.489, 45.705) -> (-11.489, 45.6034) centre (-11.489, 45.6542) ccw
  line L261 (-9.711, 45.6542) -> (-9.711, 41.9458)
  arc A798 (-9.7618, 41.9458) -> (-9.6602, 41.9458) centre (-9.711, 41.9458) ccw
  arc A799 (-9.6602, 45.6542) -> (-9.7618, 45.6542) centre (-9.711, 45.6542) ccw
  line L262 (-9.711, 41.9458) -> (-11.489, 41.9458)
  arc A800 (-11.489, 41.9966) -> (-11.489, 41.895) centre (-11.489, 41.9458) ccw
  arc A801 (-9.711, 41.895) -> (-9.711, 41.9966) centre (-9.711, 41.9458) ccw
  arc A802 (-23.984, 43.0412) -> (-23.984, 43.1428) centre (-23.984, 43.092) ccw
  line L263 (-4.084, 40.692) -> (-6.116, 40.692)
  arc A803 (-6.116, 40.7428) -> (-6.116, 40.6412) centre (-6.116, 40.692) ccw
  arc A804 (-4.084, 40.6412) -> (-4.084, 40.7428) centre (-4.084, 40.692) ccw
  line L264 (-6.116, 40.692) -> (-6.116, 41.708)
  arc A805 (-6.0652, 41.708) -> (-6.1668, 41.708) centre (-6.116, 41.708) ccw
  arc A806 (-6.1668, 40.692) -> (-6.0652, 40.692) centre (-6.116, 40.692) ccw
  line L265 (-6.116, 41.708) -> (-4.084, 41.708)
  arc A807 (-4.084, 41.6572) -> (-4.084, 41.7588) centre (-4.084, 41.708) ccw
  arc A808 (-6.116, 41.7588) -> (-6.116, 41.6572) centre (-6.116, 41.708) ccw
  line L266 (-4.084, 41.708) -> (-4.084, 40.692)
  arc A809 (-4.1348, 40.692) -> (-4.0332, 40.692) centre (-4.084, 40.692) ccw
  arc A810 (-4.0332, 41.708) -> (-4.1348, 41.708) centre (-4.084, 41.708) ccw
  line L267 (-26.016, 43.092) -> (-26.016, 44.108)
  line L268 (-8.335, 38.603) -> (-8.335, 41.397)
  arc A811 (-8.2842, 41.397) -> (-8.3858, 41.397) centre (-8.335, 41.397) ccw
  arc A812 (-8.3858, 38.603) -> (-8.2842, 38.603) centre (-8.335, 38.603) ccw
  line L269 (-8.335, 41.397) -> (-7.065, 41.397)
  arc A813 (-7.065, 41.3462) -> (-7.065, 41.4478) centre (-7.065, 41.397) ccw
  arc A814 (-8.335, 41.4478) -> (-8.335, 41.3462) centre (-8.335, 41.397) ccw
  line L270 (-7.065, 41.397) -> (-7.065, 38.603)
  arc A815 (-7.1158, 38.603) -> (-7.0142, 38.603) centre (-7.065, 38.603) ccw
  arc A816 (-7.0142, 41.397) -> (-7.1158, 41.397) centre (-7.065, 41.397) ccw
  line L271 (-7.065, 38.603) -> (-8.335, 38.603)
  arc A817 (-8.335, 38.6538) -> (-8.335, 38.5522) centre (-8.335, 38.603) ccw
  arc A818 (-7.065, 38.5522) -> (-7.065, 38.6538) centre (-7.065, 38.603) ccw
  arc A819 (-25.9652, 44.108) -> (-26.0668, 44.108) centre (-26.016, 44.108) ccw
  line L272 (-8.703, 37.565) -> (-11.497, 37.565)
  arc A820 (-11.497, 37.6158) -> (-11.497, 37.5142) centre (-11.497, 37.565) ccw
  arc A821 (-8.703, 37.5142) -> (-8.703, 37.6158) centre (-8.703, 37.565) ccw
  line L273 (-11.497, 37.565) -> (-11.497, 38.835)
  arc A822 (-11.4462, 38.835) -> (-11.5478, 38.835) centre (-11.497, 38.835) ccw
  arc A823 (-11.5478, 37.565) -> (-11.4462, 37.565) centre (-11.497, 37.565) ccw
  line L274 (-11.497, 38.835) -> (-8.703, 38.835)
  arc A824 (-8.703, 38.7842) -> (-8.703, 38.8858) centre (-8.703, 38.835) ccw
  arc A825 (-11.497, 38.8858) -> (-11.497, 38.7842) centre (-11.497, 38.835) ccw
  line L275 (-8.703, 38.835) -> (-8.703, 37.565)
  arc A826 (-8.7538, 37.565) -> (-8.6522, 37.565) centre (-8.703, 37.565) ccw
  arc A827 (-8.6522, 38.835) -> (-8.7538, 38.835) centre (-8.703, 38.835) ccw
  arc A828 (-26.0668, 43.092) -> (-25.9652, 43.092) centre (-26.016, 43.092) ccw
  line L276 (-3.589, 43.5458) -> (-3.589, 47.2542)
  arc A829 (-3.5382, 47.2542) -> (-3.6398, 47.2542) centre (-3.589, 47.2542) ccw
  arc A830 (-3.6398, 43.5458) -> (-3.5382, 43.5458) centre (-3.589, 43.5458) ccw
  line L277 (-3.589, 47.2542) -> (-1.811, 47.2542)
  arc A831 (-1.811, 47.2034) -> (-1.811, 47.305) centre (-1.811, 47.2542) ccw
  arc A832 (-3.589, 47.305) -> (-3.589, 47.2034) centre (-3.589, 47.2542) ccw
  line L278 (-1.811, 47.2542) -> (-1.811, 43.5458)
  arc A833 (-1.8618, 43.5458) -> (-1.7602, 43.5458) centre (-1.811, 43.5458) ccw
  arc A834 (-1.7602, 47.2542) -> (-1.8618, 47.2542) centre (-1.811, 47.2542) ccw
  line L279 (-1.811, 43.5458) -> (-3.589, 43.5458)
  arc A835 (-3.589, 43.5966) -> (-3.589, 43.495) centre (-3.589, 43.5458) ccw
  arc A836 (-1.811, 43.495) -> (-1.811, 43.5966) centre (-1.811, 43.5458) ccw
  line L280 (-40.9458, -38.389) -> (-44.6542, -38.389)
  line L281 (2.797, -90.335) -> (0.003, -90.335)
  arc A837 (0.003, -90.2842) -> (0.003, -90.3858) centre (0.003, -90.335) ccw
  arc A838 (2.797, -90.3858) -> (2.797, -90.2842) centre (2.797, -90.335) ccw
  line L282 (0.003, -90.335) -> (0.003, -89.065)
  arc A839 (0.0538, -89.065) -> (-0.0478, -89.065) centre (0.003, -89.065) ccw
  arc A840 (-0.0478, -90.335) -> (0.0538, -90.335) centre (0.003, -90.335) ccw
  line L283 (0.003, -89.065) -> (2.797, -89.065)
  arc A841 (2.797, -89.1158) -> (2.797, -89.0142) centre (2.797, -89.065) ccw
  arc A842 (0.003, -89.0142) -> (0.003, -89.1158) centre (0.003, -89.065) ccw
  line L284 (2.797, -89.065) -> (2.797, -90.335)
  arc A843 (2.7462, -90.335) -> (2.8478, -90.335) centre (2.797, -90.335) ccw
  arc A844 (2.8478, -89.065) -> (2.7462, -89.065) centre (2.797, -89.065) ccw
  arc A845 (-44.6542, -38.3382) -> (-44.6542, -38.4398) centre (-44.6542, -38.389) ccw
  line L285 (-0.392, -88.984) -> (-0.392, -91.016)
  arc A846 (-0.4428, -91.016) -> (-0.3412, -91.016) centre (-0.392, -91.016) ccw
  arc A847 (-0.3412, -88.984) -> (-0.4428, -88.984) centre (-0.392, -88.984) ccw
  line L286 (-0.392, -91.016) -> (-1.408, -91.016)
  arc A848 (-1.408, -90.9652) -> (-1.408, -91.0668) centre (-1.408, -91.016) ccw
  arc A849 (-0.392, -91.0668) -> (-0.392, -90.9652) centre (-0.392, -91.016) ccw
  line L287 (-1.408, -91.016) -> (-1.408, -88.984)
  arc A850 (-1.3572, -88.984) -> (-1.4588, -88.984) centre (-1.408, -88.984) ccw
  arc A851 (-1.4588, -91.016) -> (-1.3572, -91.016) centre (-1.408, -91.016) ccw
  line L288 (-1.408, -88.984) -> (-0.392, -88.984)
  arc A852 (-0.392, -89.0348) -> (-0.392, -88.9332) centre (-0.392, -88.984) ccw
  arc A853 (-1.408, -88.9332) -> (-1.408, -89.0348) centre (-1.408, -88.984) ccw
  arc A854 (-40.9458, -38.4398) -> (-40.9458, -38.3382) centre (-40.9458, -38.389) ccw
  line L289 (2.797, -92.035) -> (0.003, -92.035)
  arc A855 (0.003, -91.9842) -> (0.003, -92.0858) centre (0.003, -92.035) ccw
  arc A856 (2.797, -92.0858) -> (2.797, -91.9842) centre (2.797, -92.035) ccw
  line L290 (0.003, -92.035) -> (0.003, -90.765)
  arc A857 (0.0538, -90.765) -> (-0.0478, -90.765) centre (0.003, -90.765) ccw
  arc A858 (-0.0478, -92.035) -> (0.0538, -92.035) centre (0.003, -92.035) ccw
  line L291 (0.003, -90.765) -> (2.797, -90.765)
  arc A859 (2.797, -90.8158) -> (2.797, -90.7142) centre (2.797, -90.765) ccw
  arc A860 (0.003, -90.7142) -> (0.003, -90.8158) centre (0.003, -90.765) ccw
  line L292 (2.797, -90.765) -> (2.797, -92.035)
  arc A861 (2.7462, -92.035) -> (2.8478, -92.035) centre (2.797, -92.035) ccw
  arc A862 (2.8478, -90.765) -> (2.7462, -90.765) centre (2.797, -90.765) ccw
  line L293 (-44.6542, -38.389) -> (-44.6542, -36.611)
  line L294 (-12.103, 9.065) -> (-14.897, 9.065)
  arc A863 (-14.897, 9.1158) -> (-14.897, 9.0142) centre (-14.897, 9.065) ccw
  arc A864 (-12.103, 9.0142) -> (-12.103, 9.1158) centre (-12.103, 9.065) ccw
  line L295 (-14.897, 9.065) -> (-14.897, 10.335)
  arc A865 (-14.8462, 10.335) -> (-14.9478, 10.335) centre (-14.897, 10.335) ccw
  arc A866 (-14.9478, 9.065) -> (-14.8462, 9.065) centre (-14.897, 9.065) ccw
  line L296 (-14.897, 10.335) -> (-12.103, 10.335)
  arc A867 (-12.103, 10.2842) -> (-12.103, 10.3858) centre (-12.103, 10.335) ccw
  arc A868 (-14.897, 10.3858) -> (-14.897, 10.2842) centre (-14.897, 10.335) ccw
  line L297 (-12.103, 10.335) -> (-12.103, 9.065)
  arc A869 (-12.1538, 9.065) -> (-12.0522, 9.065) centre (-12.103, 9.065) ccw
  arc A870 (-12.0522, 10.335) -> (-12.1538, 10.335) centre (-12.103, 10.335) ccw
  arc A871 (-44.6034, -36.611) -> (-44.705, -36.611) centre (-44.6542, -36.611) ccw
  line L298 (-4.984, 8.192) -> (-7.016, 8.192)
  arc A872 (-7.016, 8.2428) -> (-7.016, 8.1412) centre (-7.016, 8.192) ccw
  arc A873 (-4.984, 8.1412) -> (-4.984, 8.2428) centre (-4.984, 8.192) ccw
  line L299 (-7.016, 8.192) -> (-7.016, 9.208)
  arc A874 (-6.9652, 9.208) -> (-7.0668, 9.208) centre (-7.016, 9.208) ccw
  arc A875 (-7.0668, 8.192) -> (-6.9652, 8.192) centre (-7.016, 8.192) ccw
  line L300 (-7.016, 9.208) -> (-4.984, 9.208)
  arc A876 (-4.984, 9.1572) -> (-4.984, 9.2588) centre (-4.984, 9.208) ccw
  arc A877 (-7.016, 9.2588) -> (-7.016, 9.1572) centre (-7.016, 9.208) ccw
  line L301 (-4.984, 9.208) -> (-4.984, 8.192)
  arc A878 (-5.0348, 8.192) -> (-4.9332, 8.192) centre (-4.984, 8.192) ccw
  arc A879 (-4.9332, 9.208) -> (-5.0348, 9.208) centre (-4.984, 9.208) ccw
  arc A880 (-44.705, -38.389) -> (-44.6034, -38.389) centre (-44.6542, -38.389) ccw
  line L302 (-7.176, 22.113) -> (-7.176, 17.287)
  arc A881 (-7.2268, 17.287) -> (-7.1252, 17.287) centre (-7.176, 17.287) ccw
  arc A882 (-7.1252, 22.113) -> (-7.2268, 22.113) centre (-7.176, 22.113) ccw
  line L303 (-7.176, 17.287) -> (-10.224, 17.287)
  arc A883 (-10.224, 17.3378) -> (-10.224, 17.2362) centre (-10.224, 17.287) ccw
  arc A884 (-7.176, 17.2362) -> (-7.176, 17.3378) centre (-7.176, 17.287) ccw
  line L304 (-10.224, 17.287) -> (-10.224, 22.113)
  arc A885 (-10.1732, 22.113) -> (-10.2748, 22.113) centre (-10.224, 22.113) ccw
  arc A886 (-10.2748, 17.287) -> (-10.1732, 17.287) centre (-10.224, 17.287) ccw
  line L305 (-10.224, 22.113) -> (-7.176, 22.113)
  arc A887 (-7.176, 22.0622) -> (-7.176, 22.1638) centre (-7.176, 22.113) ccw
  arc A888 (-10.224, 22.1638) -> (-10.224, 22.0622) centre (-10.224, 22.113) ccw
  line L306 (-44.6542, -36.611) -> (-40.9458, -36.611)
  line L307 (-10.211, 21.0542) -> (-10.211, 17.3458)
  arc A889 (-10.2618, 17.3458) -> (-10.1602, 17.3458) centre (-10.211, 17.3458) ccw
  arc A890 (-10.1602, 21.0542) -> (-10.2618, 21.0542) centre (-10.211, 21.0542) ccw
  line L308 (-10.211, 17.3458) -> (-11.989, 17.3458)
  arc A891 (-11.989, 17.3966) -> (-11.989, 17.295) centre (-11.989, 17.3458) ccw
  arc A892 (-10.211, 17.295) -> (-10.211, 17.3966) centre (-10.211, 17.3458) ccw
  line L309 (-11.989, 17.3458) -> (-11.989, 21.0542)
  arc A893 (-11.9382, 21.0542) -> (-12.0398, 21.0542) centre (-11.989, 21.0542) ccw
  arc A894 (-12.0398, 17.3458) -> (-11.9382, 17.3458) centre (-11.989, 17.3458) ccw
  line L310 (-11.989, 21.0542) -> (-10.211, 21.0542)
  arc A895 (-10.211, 21.0034) -> (-10.211, 21.105) centre (-10.211, 21.0542) ccw
  arc A896 (-11.989, 21.105) -> (-11.989, 21.0034) centre (-11.989, 21.0542) ccw
  arc A897 (-40.9458, -36.6618) -> (-40.9458, -36.5602) centre (-40.9458, -36.611) ccw
  line L311 (-14.889, 10.3458) -> (-14.889, 14.0542)
  arc A898 (-14.8382, 14.0542) -> (-14.9398, 14.0542) centre (-14.889, 14.0542) ccw
  arc A899 (-14.9398, 10.3458) -> (-14.8382, 10.3458) centre (-14.889, 10.3458) ccw
  line L312 (-14.889, 14.0542) -> (-13.111, 14.0542)
  arc A900 (-13.111, 14.0034) -> (-13.111, 14.105) centre (-13.111, 14.0542) ccw
  arc A901 (-14.889, 14.105) -> (-14.889, 14.0034) centre (-14.889, 14.0542) ccw
  line L313 (-13.111, 14.0542) -> (-13.111, 10.3458)
  arc A902 (-13.1618, 10.3458) -> (-13.0602, 10.3458) centre (-13.111, 10.3458) ccw
  arc A903 (-13.0602, 14.0542) -> (-13.1618, 14.0542) centre (-13.111, 14.0542) ccw
  line L314 (-13.111, 10.3458) -> (-14.889, 10.3458)
  arc A904 (-14.889, 10.3966) -> (-14.889, 10.295) centre (-14.889, 10.3458) ccw
  arc A905 (-13.111, 10.295) -> (-13.111, 10.3966) centre (-13.111, 10.3458) ccw
  arc A906 (-44.6542, -36.5602) -> (-44.6542, -36.6618) centre (-44.6542, -36.611) ccw
  line L315 (-19.111, 5.0542) -> (-19.111, 1.3458)
  arc A907 (-19.1618, 1.3458) -> (-19.0602, 1.3458) centre (-19.111, 1.3458) ccw
  arc A908 (-19.0602, 5.0542) -> (-19.1618, 5.0542) centre (-19.111, 5.0542) ccw
  line L316 (-19.111, 1.3458) -> (-20.889, 1.3458)
  arc A909 (-20.889, 1.3966) -> (-20.889, 1.295) centre (-20.889, 1.3458) ccw
  arc A910 (-19.111, 1.295) -> (-19.111, 1.3966) centre (-19.111, 1.3458) ccw
  line L317 (-20.889, 1.3458) -> (-20.889, 5.0542)
  arc A911 (-20.8382, 5.0542) -> (-20.9398, 5.0542) centre (-20.889, 5.0542) ccw
  arc A912 (-20.9398, 1.3458) -> (-20.8382, 1.3458) centre (-20.889, 1.3458) ccw
  line L318 (-20.889, 5.0542) -> (-19.111, 5.0542)
  arc A913 (-19.111, 5.0034) -> (-19.111, 5.105) centre (-19.111, 5.0542) ccw
  arc A914 (-20.889, 5.105) -> (-20.889, 5.0034) centre (-20.889, 5.0542) ccw
  line L319 (-40.9458, -36.611) -> (-40.9458, -38.389)
  line L320 (-9.111, 16.0542) -> (-9.111, 12.3458)
  arc A915 (-9.1618, 12.3458) -> (-9.0602, 12.3458) centre (-9.111, 12.3458) ccw
  arc A916 (-9.0602, 16.0542) -> (-9.1618, 16.0542) centre (-9.111, 16.0542) ccw
  line L321 (-9.111, 12.3458) -> (-10.889, 12.3458)
  arc A917 (-10.889, 12.3966) -> (-10.889, 12.295) centre (-10.889, 12.3458) ccw
  arc A918 (-9.111, 12.295) -> (-9.111, 12.3966) centre (-9.111, 12.3458) ccw
  line L322 (-10.889, 12.3458) -> (-10.889, 16.0542)
  arc A919 (-10.8382, 16.0542) -> (-10.9398, 16.0542) centre (-10.889, 16.0542) ccw
  arc A920 (-10.9398, 12.3458) -> (-10.8382, 12.3458) centre (-10.889, 12.3458) ccw
  line L323 (-10.889, 16.0542) -> (-9.111, 16.0542)
  arc A921 (-9.111, 16.0034) -> (-9.111, 16.105) centre (-9.111, 16.0542) ccw
  arc A922 (-10.889, 16.105) -> (-10.889, 16.0034) centre (-10.889, 16.0542) ccw
  arc A923 (-40.9966, -38.389) -> (-40.895, -38.389) centre (-40.9458, -38.389) ccw
  line L324 (-5.992, 5.216) -> (-5.992, 3.184)
  arc A924 (-6.0428, 3.184) -> (-5.9412, 3.184) centre (-5.992, 3.184) ccw
  arc A925 (-5.9412, 5.216) -> (-6.0428, 5.216) centre (-5.992, 5.216) ccw
  line L325 (-5.992, 3.184) -> (-7.008, 3.184)
  arc A926 (-7.008, 3.2348) -> (-7.008, 3.1332) centre (-7.008, 3.184) ccw
  arc A927 (-5.992, 3.1332) -> (-5.992, 3.2348) centre (-5.992, 3.184) ccw
  line L326 (-7.008, 3.184) -> (-7.008, 5.216)
  arc A928 (-6.9572, 5.216) -> (-7.0588, 5.216) centre (-7.008, 5.216) ccw
  arc A929 (-7.0588, 3.184) -> (-6.9572, 3.184) centre (-7.008, 3.184) ccw
  line L327 (-7.008, 5.216) -> (-5.992, 5.216)
  arc A930 (-5.992, 5.1652) -> (-5.992, 5.2668) centre (-5.992, 5.216) ccw
  arc A931 (-7.008, 5.2668) -> (-7.008, 5.1652) centre (-7.008, 5.216) ccw
  arc A932 (-40.895, -36.611) -> (-40.9966, -36.611) centre (-40.9458, -36.611) ccw
  line L328 (-16.008, -6.816) -> (-16.008, -4.784)
  arc A933 (-15.9572, -4.784) -> (-16.0588, -4.784) centre (-16.008, -4.784) ccw
  arc A934 (-16.0588, -6.816) -> (-15.9572, -6.816) centre (-16.008, -6.816) ccw
  line L329 (-16.008, -4.784) -> (-14.992, -4.784)
  arc A935 (-14.992, -4.8348) -> (-14.992, -4.7332) centre (-14.992, -4.784) ccw
  arc A936 (-16.008, -4.7332) -> (-16.008, -4.8348) centre (-16.008, -4.784) ccw
  line L330 (-14.992, -4.784) -> (-14.992, -6.816)
  arc A937 (-15.0428, -6.816) -> (-14.9412, -6.816) centre (-14.992, -6.816) ccw
  arc A938 (-14.9412, -4.784) -> (-15.0428, -4.784) centre (-14.992, -4.784) ccw
  line L331 (-14.992, -6.816) -> (-16.008, -6.816)
  arc A939 (-16.008, -6.7652) -> (-16.008, -6.8668) centre (-16.008, -6.816) ccw
  arc A940 (-14.992, -6.8668) -> (-14.992, -6.7652) centre (-14.992, -6.816) ccw
  line L332 (41.116, 47.492) -> (39.084, 47.492)
  line L333 (-12.889, 10.3458) -> (-12.889, 14.0542)
  arc A941 (-12.8382, 14.0542) -> (-12.9398, 14.0542) centre (-12.889, 14.0542) ccw
  arc A942 (-12.9398, 10.3458) -> (-12.8382, 10.3458) centre (-12.889, 10.3458) ccw
  line L334 (-12.889, 14.0542) -> (-11.111, 14.0542)
  arc A943 (-11.111, 14.0034) -> (-11.111, 14.105) centre (-11.111, 14.0542) ccw
  arc A944 (-12.889, 14.105) -> (-12.889, 14.0034) centre (-12.889, 14.0542) ccw
  line L335 (-11.111, 14.0542) -> (-11.111, 10.3458)
  arc A945 (-11.1618, 10.3458) -> (-11.0602, 10.3458) centre (-11.111, 10.3458) ccw
  arc A946 (-11.0602, 14.0542) -> (-11.1618, 14.0542) centre (-11.111, 14.0542) ccw
  line L336 (-11.111, 10.3458) -> (-12.889, 10.3458)
  arc A947 (-12.889, 10.3966) -> (-12.889, 10.295) centre (-12.889, 10.3458) ccw
  arc A948 (-11.111, 10.295) -> (-11.111, 10.3966) centre (-11.111, 10.3458) ccw
  arc A949 (39.084, 47.5428) -> (39.084, 47.4412) centre (39.084, 47.492) ccw
  line L337 (-6.992, 5.216) -> (-6.992, 3.184)
  arc A950 (-7.0428, 3.184) -> (-6.9412, 3.184) centre (-6.992, 3.184) ccw
  arc A951 (-6.9412, 5.216) -> (-7.0428, 5.216) centre (-6.992, 5.216) ccw
  line L338 (-6.992, 3.184) -> (-8.008, 3.184)
  arc A952 (-8.008, 3.2348) -> (-8.008, 3.1332) centre (-8.008, 3.184) ccw
  arc A953 (-6.992, 3.1332) -> (-6.992, 3.2348) centre (-6.992, 3.184) ccw
  line L339 (-8.008, 3.184) -> (-8.008, 5.216)
  arc A954 (-7.9572, 5.216) -> (-8.0588, 5.216) centre (-8.008, 5.216) ccw
  arc A955 (-8.0588, 3.184) -> (-7.9572, 3.184) centre (-8.008, 3.184) ccw
  line L340 (-8.008, 5.216) -> (-6.992, 5.216)
  arc A956 (-6.992, 5.1652) -> (-6.992, 5.2668) centre (-6.992, 5.216) ccw
  arc A957 (-8.008, 5.2668) -> (-8.008, 5.1652) centre (-8.008, 5.216) ccw
  arc A958 (41.116, 47.4412) -> (41.116, 47.5428) centre (41.116, 47.492) ccw
  line L341 (-10.992, -8.784) -> (-10.992, -10.816)
  arc A959 (-11.0428, -10.816) -> (-10.9412, -10.816) centre (-10.992, -10.816) ccw
  arc A960 (-10.9412, -8.784) -> (-11.0428, -8.784) centre (-10.992, -8.784) ccw
  line L342 (-10.992, -10.816) -> (-12.008, -10.816)
  arc A961 (-12.008, -10.7652) -> (-12.008, -10.8668) centre (-12.008, -10.816) ccw
  arc A962 (-10.992, -10.8668) -> (-10.992, -10.7652) centre (-10.992, -10.816) ccw
  line L343 (-12.008, -10.816) -> (-12.008, -8.784)
  arc A963 (-11.9572, -8.784) -> (-12.0588, -8.784) centre (-12.008, -8.784) ccw
  arc A964 (-12.0588, -10.816) -> (-11.9572, -10.816) centre (-12.008, -10.816) ccw
  line L344 (-12.008, -8.784) -> (-10.992, -8.784)
  arc A965 (-10.992, -8.8348) -> (-10.992, -8.7332) centre (-10.992, -8.784) ccw
  arc A966 (-12.008, -8.7332) -> (-12.008, -8.8348) centre (-12.008, -8.784) ccw
  line L345 (39.084, 47.492) -> (39.084, 48.508)
  line L346 (-12.992, -4.784) -> (-12.992, -6.816)
  arc A967 (-13.0428, -6.816) -> (-12.9412, -6.816) centre (-12.992, -6.816) ccw
  arc A968 (-12.9412, -4.784) -> (-13.0428, -4.784) centre (-12.992, -4.784) ccw
  line L347 (-12.992, -6.816) -> (-14.008, -6.816)
  arc A969 (-14.008, -6.7652) -> (-14.008, -6.8668) centre (-14.008, -6.816) ccw
  arc A970 (-12.992, -6.8668) -> (-12.992, -6.7652) centre (-12.992, -6.816) ccw
  line L348 (-14.008, -6.816) -> (-14.008, -4.784)
  arc A971 (-13.9572, -4.784) -> (-14.0588, -4.784) centre (-14.008, -4.784) ccw
  arc A972 (-14.0588, -6.816) -> (-13.9572, -6.816) centre (-14.008, -6.816) ccw
  line L349 (-14.008, -4.784) -> (-12.992, -4.784)
  arc A973 (-12.992, -4.8348) -> (-12.992, -4.7332) centre (-12.992, -4.784) ccw
  arc A974 (-14.008, -4.7332) -> (-14.008, -4.8348) centre (-14.008, -4.784) ccw
  arc A975 (39.1348, 48.508) -> (39.0332, 48.508) centre (39.084, 48.508) ccw
  line L350 (-3.897, 4.835) -> (-1.103, 4.835)
  arc A976 (-1.103, 4.7842) -> (-1.103, 4.8858) centre (-1.103, 4.835) ccw
  arc A977 (-3.897, 4.8858) -> (-3.897, 4.7842) centre (-3.897, 4.835) ccw
  line L351 (-1.103, 4.835) -> (-1.103, 3.565)
  arc A978 (-1.1538, 3.565) -> (-1.0522, 3.565) centre (-1.103, 3.565) ccw
  arc A979 (-1.0522, 4.835) -> (-1.1538, 4.835) centre (-1.103, 4.835) ccw
  line L352 (-1.103, 3.565) -> (-3.897, 3.565)
  arc A980 (-3.897, 3.6158) -> (-3.897, 3.5142) centre (-3.897, 3.565) ccw
  arc A981 (-1.103, 3.5142) -> (-1.103, 3.6158) centre (-1.103, 3.565) ccw
  line L353 (-3.897, 3.565) -> (-3.897, 4.835)
  arc A982 (-3.8462, 4.835) -> (-3.9478, 4.835) centre (-3.897, 4.835) ccw
  arc A983 (-3.9478, 3.565) -> (-3.8462, 3.565) centre (-3.897, 3.565) ccw
  arc A984 (39.0332, 47.492) -> (39.1348, 47.492) centre (39.084, 47.492) ccw
  line L354 (-8.992, 7.216) -> (-8.992, 5.184)
  arc A985 (-9.0428, 5.184) -> (-8.9412, 5.184) centre (-8.992, 5.184) ccw
  arc A986 (-8.9412, 7.216) -> (-9.0428, 7.216) centre (-8.992, 7.216) ccw
  line L355 (-8.992, 5.184) -> (-10.008, 5.184)
  arc A987 (-10.008, 5.2348) -> (-10.008, 5.1332) centre (-10.008, 5.184) ccw
  arc A988 (-8.992, 5.1332) -> (-8.992, 5.2348) centre (-8.992, 5.184) ccw
  line L356 (-10.008, 5.184) -> (-10.008, 7.216)
  arc A989 (-9.9572, 7.216) -> (-10.0588, 7.216) centre (-10.008, 7.216) ccw
  arc A990 (-10.0588, 5.184) -> (-9.9572, 5.184) centre (-10.008, 5.184) ccw
  line L357 (-10.008, 7.216) -> (-8.992, 7.216)
  arc A991 (-8.992, 7.1652) -> (-8.992, 7.2668) centre (-8.992, 7.216) ccw
  arc A992 (-10.008, 7.2668) -> (-10.008, 7.1652) centre (-10.008, 7.216) ccw
  line L358 (39.084, 48.508) -> (41.116, 48.508)
  line L359 (1.992, 6.184) -> (1.992, 8.216)
  arc A993 (2.0428, 8.216) -> (1.9412, 8.216) centre (1.992, 8.216) ccw
  arc A994 (1.9412, 6.184) -> (2.0428, 6.184) centre (1.992, 6.184) ccw
  line L360 (1.992, 8.216) -> (3.008, 8.216)
  arc A995 (3.008, 8.1652) -> (3.008, 8.2668) centre (3.008, 8.216) ccw
  arc A996 (1.992, 8.2668) -> (1.992, 8.1652) centre (1.992, 8.216) ccw
  line L361 (3.008, 8.216) -> (3.008, 6.184)
  arc A997 (2.9572, 6.184) -> (3.0588, 6.184) centre (3.008, 6.184) ccw
  arc A998 (3.0588, 8.216) -> (2.9572, 8.216) centre (3.008, 8.216) ccw
  line L362 (3.008, 6.184) -> (1.992, 6.184)
  arc A999 (1.992, 6.2348) -> (1.992, 6.1332) centre (1.992, 6.184) ccw
  arc A1000 (3.008, 6.1332) -> (3.008, 6.2348) centre (3.008, 6.184) ccw
  arc A1001 (41.116, 48.4572) -> (41.116, 48.5588) centre (41.116, 48.508) ccw
  line L363 (-4.016, 13.208) -> (-1.984, 13.208)
  arc A1002 (-1.984, 13.1572) -> (-1.984, 13.2588) centre (-1.984, 13.208) ccw
  arc A1003 (-4.016, 13.2588) -> (-4.016, 13.1572) centre (-4.016, 13.208) ccw
  line L364 (-1.984, 13.208) -> (-1.984, 12.192)
  arc A1004 (-2.0348, 12.192) -> (-1.9332, 12.192) centre (-1.984, 12.192) ccw
  arc A1005 (-1.9332, 13.208) -> (-2.0348, 13.208) centre (-1.984, 13.208) ccw
  line L365 (-1.984, 12.192) -> (-4.016, 12.192)
  arc A1006 (-4.016, 12.2428) -> (-4.016, 12.1412) centre (-4.016, 12.192) ccw
  arc A1007 (-1.984, 12.1412) -> (-1.984, 12.2428) centre (-1.984, 12.192) ccw